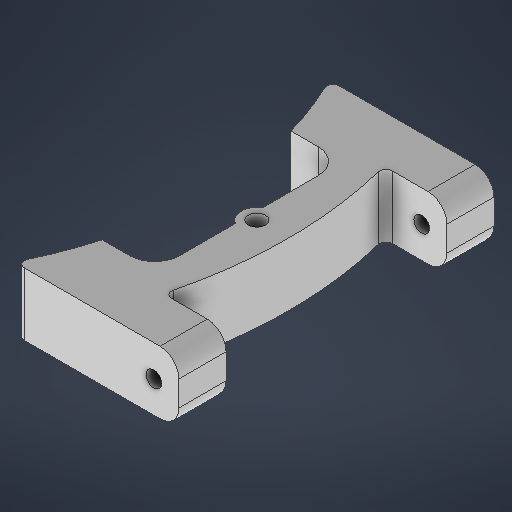
# Autodesk Inventor part: Cylinder 80-20 Spacer_1 Slant
Saved by Autodesk Inventor 2025 (Build 290162000, 162)
## iProperties
Created: 2024-04-28
Part Number: Cylinder 80-20 Spacer_1 Slant
Material: Generic
Document SubType Name: Modeling
Designer: Thienan Hoang
Density: 1 g/cm^3
Appearance: Default
Author: Thienan Hoang
Autodesk Inventor part; units mm, degrees
note: some values were not read from the file. Chosen so that the rebuilt part matches the saved one: direction of "Hole2".
ref_plane "YZ Plane" through (0, 0, 0) normal (1, 0, 0) x (0, 1, 0)
ref_plane "XZ Plane" through (0, 0, 0) normal (0, 1, 0) x (-1, 0, 0)
ref_plane "XY Plane" through (0, 0, 0) normal (0, 0, 1) x (1, 0, 0)
sketch "Sketch1" plane through (0, 0, 0) normal (0, 1, 0) x (-1, 0, 0)
  circle A0 centre (0, 0) radius 135
  circle A1 centre (0, 0) radius 110
  line L0 (0, 0) -> (-125, 0)
  line L1 (0, 0) -> (125, 0) construction
  circle A2 centre (-125, 0) radius 2.75
  circle A3 centre (-125, 0) radius 5
  dimension "d0" = 270
  dimension "d1" = 220
  dimension "d82" = 125
  dimension "d83" = 180
  dimension "d84" = 5.5
  dimension "d85" = 10
  constraints: 4 centre point, 4 coincident, 4 end point, 2 horizontal, 1 collinear
  measures "d0" diameter of A0
  measures "d1" diameter of A1
  measures "d82" distance of L0.start L0.end
  measures "d83" angle of L0 L1
  measures "d84" diameter of A2
  measures "d85" diameter of A3
extrude "Extrusion1" add sketch "Sketch1" along normal mid plane 20 contours A0 | A2 | A3
sketch "Sketch4" plane through (0, 10, 0) normal (0, 1, 0) x (1, 0, 0)
  circle A0 centre (0, 0) radius 50.125
  circle A1 centre (0, 0) radius 135 projected
  circle A2 centre (0, 0) radius 110 projected
  line L0 (125.3494, 50.125) -> (150.3494, 50.125)
  line L1 (150.3494, 50.125) -> (150.3494, 35.125)
  line L2 (150.3494, 35.125) -> (125.3494, 35.125)
  line L3 (125.3494, 35.125) -> (125.3494, 50.125)
  line L4 (150.3494, 70.125) -> (104.7795, 70.125)
  line L5 (104.7795, 70.125) -> (104.7795, 85.125)
  line L6 (104.7795, 85.125) -> (150.3494, 85.125)
  line L7 (150.3494, 85.125) -> (150.3494, 70.125)
  line L8 (103.1497, 60.125) -> (138.3886, 60.125) construction
  point P0 (130.3504, 35.125)
  point P1 (115.3581, 70.125)
  dimension "d21" = 100.25
  dimension "d22" = 25
  dimension "d23" = 15
  dimension "d24" = 20
  dimension "d25" = 15
  dimension "d57" = 10
  constraints: 18 end point, 4 parallel, 3 horizontal, 2 perpendicular, 2 point on circle, 1 centre point, 1 coincident, 1 collinear, 1 other
  measures "d21" diameter of A0
  measures "d22" distance of L1.end L2.end
  measures "d23" distance of L0.end L1.end
  measures "d24" distance between parallel lines of L0 L4
  measures "d25" distance of L6.end L4.start
  measures "d57" distance edge to line of A0 L8
extrude "Extrusion3" add sketch "Sketch4" against normal up to surface (20 mm away) contours L6 L7 L4 A1 | A1 L0 L1 L2
fillet "Fillet1" radius 6 4 edges at (150.3494, 10, -77.625) (150.3494, -10, -77.625) (150.3494, -10, -42.625) (150.3494, 10, -42.625)
fillet "Fillet2" radius 10 1 edges at (104.7795, 0, -85.125)
fillet "Fillet3" radius 2 1 edges at (130.3504, 0, -35.125)
sketch "Sketch5" plane through (150.3494, -4, -85.125) normal (0, 0, -1) x (-1, 0, 0)
  line L0 (0, 8) -> (0, 0) projected
  line L1 (40.9135, -6) -> (6, -6) projected
  point P0 (150.3494, 4)
  point P1 (8, 4)
  point P2 (0, 4)
  dimension "d38" = 8
  dimension "d39" = 10
  constraints: 1 midpoint
  measures "d38" distance of point (0, 4) point (8, 4)
  measures "d39" distance from line of L1 point (8, 4)
hole "Hole2" at (142.3494, 0, -85.125) direction (0, 0, 1) diameter 5 depth 50 counterbore diameter 8.5 counterbore depth 5
mirror "Mirror1" about plane through (0, 0, 0) normal (1, 0, 0) of "Extrusion3", "Fillet1", "Fillet2", "Fillet3", "Hole2"
mirror "Mirror2" about plane through (0, 0, 0) normal (0, 0, 1) of "Extrusion3", "Fillet1", "Fillet2", "Fillet3", "Hole2"
sketch "Sketch10" plane through (0, 10, 0) normal (0, 1, 0) x (1, 0, 0)
  line L0 (144.3494, 50.125) -> (125.3494, 50.125) projected
  line L1 (144.3494, -50.125) -> (125.3494, -50.125) projected
  line L2 (174.7146, 50.125) -> (75.699, 50.125)
  line L3 (75.699, 50.125) -> (75.699, -50.125)
  line L4 (75.699, -50.125) -> (174.7146, -50.125)
  line L5 (174.7146, 145.3293) -> (-157.7861, 145.3293)
  line L6 (-157.7861, 145.3293) -> (-157.7861, -141.1771)
  line L7 (-157.7861, -141.1771) -> (174.7146, -141.1771)
  line L8 (174.7146, -141.1771) -> (174.7146, -50.125)
  line L9 (174.7146, 50.125) -> (174.7146, 145.3293)
  point P0 (0, 0)
  constraints: 16 end point, 4 parallel, 2 horizontal, 2 perpendicular
extrude "Extrusion7" cut sketch "Sketch10" against normal through all
fillet "Fillet7" radius 2 2 edges at (97.9157, 0, -50.125) (97.9157, 0, 50.125)
sketch "Sketch12" plane through (0, 10, 0) normal (0, 1, 0) x (1, 0, 0)
  circle A0 centre (0, 0) radius 110
  line L0 (122.5, 30) -> (97.5, 30)
  line L1 (97.5, 30) -> (97.5, -30)
  line L2 (97.5, -30) -> (122.5, -30)
  line L3 (122.5, -30) -> (122.5, 30)
  line L4 (122.5, 30) -> (97.5, -30) construction
  line L5 (97.5, 30) -> (122.5, -30) construction
  point P0 (110, 0)
  dimension "d68" = 25
  dimension "d69" = 60
  constraints: 12 end point, 2 midpoint, 2 parallel, 1 coincident, 1 horizontal, 1 horizontal alignment, 1 perpendicular, 2 other
  measures "d68" distance of L2.end L1.end
  measures "d69" distance of L1.end L0.end
extrude "Extrusion9" cut sketch "Sketch12" against normal up to surface (20 mm away) contours A0 L2 L1 L0 | A0 L0 L3 L2 picked at (101.6667, 0)
fillet "Fillet8" radius 8 2 edges at (122.5, 0, -30) (122.5, 0, 30)
extrude "Extrusion10" cut sketch "Sketch1" along normal mid plane 20 contours A2 | A3
extrude "Extrusion11" add sketch "Sketch1" along normal up to surface (10 mm away) contours A3
body "Solid1"
